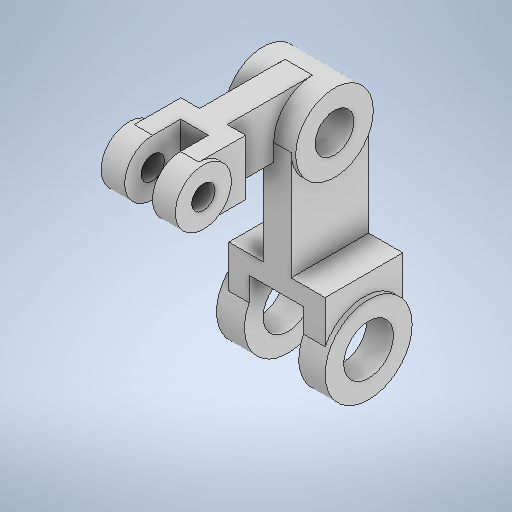
# Autodesk Inventor part: Sólido 2
Saved by Autodesk Inventor 2025 (Build 290162000, 162)
## iProperties
Created: 2024-04-28
Part Number: Sólido 2
Material: Generic
Document SubType Name: Modeling
Designer: kaike
Density: 1 g/cm^3
Appearance: Default
Author: kaike
Autodesk Inventor part; units mm, degrees
ref_plane "YZ Plane" through (0, 0, 0) normal (1, 0, 0) x (0, 1, 0)
ref_plane "XZ Plane" through (0, 0, 0) normal (0, 1, 0) x (-1, 0, 0)
sketch "Sketch1" plane through (0, 0, 0) normal (0, 0, 1) x (1, 0, 0)
  line L0 (31, 0) -> (31, 12)
  line L1 (31, 12) -> (9, 12)
  line L2 (9, 12) -> (9, 82)
  line L3 (31, 0) -> (17, 0)
  line L4 (17, 0) -> (0, 0)
  line L5 (9, 82) -> (0, 82)
  line L6 (-31, 0) -> (-31, 12)
  line L7 (-31, 12) -> (-9, 12)
  line L8 (-9, 12) -> (-9, 82)
  line L9 (-31, 0) -> (-17, 0)
  line L10 (-17, 0) -> (0, 0)
  line L11 (-9, 82) -> (0, 82)
  point P0 (0, 0)
  dimension "d7" = 14
  dimension "d8" = 17
  dimension "d10" = 70
  dimension "d11" = 22
  dimension "d12" = 12
  dimension "d13" = 18
  constraints: 24 end point, 2 horizontal
  measures "d7" distance of L0.start L3.end
  measures "d8" distance of L3.end L4.end
  measures "d10" distance of L8.start L11.start
  measures "d11" distance of L0.end L1.end
  measures "d12" distance of L0.start L0.end
  measures "d13" distance of L11.start L2.end
extrude "Extrusion1" add sketch "Sketch1" along normal mid plane 50
sketch "Sketch2" plane through (31, 0, 25) normal (1, 0, 0) x (0, 0, -1)
  line L0 (50, 82) -> (0, 82) projected
  circle A0 centre (25, -28) radius 28
  point P0 (25, 0)
  dimension "d17" = 56
  constraints: 1 centre point
  measures "d17" diameter of A0
extrude "Extrusion2" add sketch "Sketch2" along normal blind 3
sketch "Sketch3" plane through (31, 0, 25) normal (-1, 0, 0) x (0, 0, 1)
  arc A0 (-53, -28) -> (-25, 0) centre (-25, -28) ccw projected
  circle A1 centre (-25, -28) radius 28
  point P0 (-25, 0)
  constraints: 1 centre point, 1 coincident
extrude "Extrusion3" add sketch "Sketch3" along normal blind 67
sketch "Sketch5" plane through (9, 12, 25) normal (1, 0, 0) x (0, 0, -1)
  line L0 (50, 70) -> (0, 70) projected
  circle A0 centre (25, 70) radius 25
  point P0 (25, -12)
  dimension "d24" = 50
  constraints: 1 centre point, 1 midpoint
  measures "d24" diameter of A0
extrude "Extrusion5" add sketch "Sketch5" along normal blind 3
sketch "Sketch6" plane through (9, 12, 25) normal (-1, 0, 0) x (0, 0, 1)
  arc A0 (0, 70) -> (-50, 70) centre (-25, 70) ccw projected
  circle A1 centre (-25, 70) radius 25
  point P0 (-25, -12)
  point P1 (0, 70)
  constraints: 1 centre point, 1 coincident
extrude "Extrusion6" add sketch "Sketch6" along normal blind 43
sketch "Sketch7" plane through (-31, 12, 25) normal (0, 1, 0) x (1, 0, 0)
  point P0 (31, 25)
ref_plane "Work Plane1" through (12, 107, 55) normal (0, 1, 0) x (1, 0, 0)
sketch "Sketch10" plane through (12, 107, 55) normal (0, 1, 0) x (1, 0, 0)
  line L0 (-2.3312, -30.1107) -> (-2.219, -0.0002)
  line L1 (-2.219, -0.0002) -> (-14.1262, -0.0002)
  line L2 (-2.3312, -30.1107) -> (-14.238, -30.0664)
  line L3 (-44.0784, -29.9553) -> (-43.9668, 0.0445)
  line L4 (-43.9668, 0.0445) -> (-31.9669, -0.0002)
  line L5 (-44.0784, -29.9553) -> (-32.1716, -29.9996)
  line L6 (-14.1259, 55) -> (-31.9669, 55)
  line L7 (-2.219, 29.9997) -> (52.781, 29.9997) construction
  line L8 (-31.9669, -0.0002) -> (-31.9669, 55)
  line L9 (-14.1259, 55) -> (-14.1262, -0.0002)
  line L10 (-32.1716, -29.9996) -> (-14.238, -30.0664)
  constraints: 22 end point, 1 collinear, 1 horizontal, 1 perpendicular, 1 vertical
extrude "Extrusion8" add sketch "Sketch10" against normal blind 36
sketch "Sketch12" plane through (12, 82, 0) normal (1, 0, 0) x (0, 0, -1)
  circle A0 centre (0, 0) radius 12.5
  point P0 (0, -82)
  dimension "d48" = 25
  constraints: 1 centre point, 1 coincident
  measures "d48" diameter of A0
sketch "Sketch13" plane through (34, -28, 0) normal (1, 0, 0) x (0, 0, -1)
  circle A0 centre (0, 0) radius 16
  point P0 (0, 28)
  dimension "d49" = 32
  constraints: 1 centre point, 1 coincident
  measures "d49" diameter of A0
sketch "Sketch15" plane through (9.6688, 71, 85.1107) normal (1, 0, 0.0037) x (0.0037, 0, -1)
  line L0 (-0.0001, 36) -> (-0.0001, 0) projected
  circle A0 centre (-0.0001, 18) radius 18
  point P0 (85.0741, -71)
  constraints: 1 midpoint, 1 vertical alignment, 2 other
extrude "Extrusion9" add sketch "Sketch15" along normal blind 3
sketch "Sketch16" plane through (12.6688, 89, 85.1219) normal (1, 0, 0.0037) x (0.0037, 0, -1)
  circle A0 centre (0, 0) radius 18
  point P0 (85.0741, -89)
  constraints: 1 centre point
extrude "Extrusion10" add sketch "Sketch16" against normal blind 48
sketch "Sketch17" plane through (12, 107, 55) normal (0, 1, 0) x (1, 0, 0)
  line L0 (-32.1046, -11.9997) -> (-14.171, -12.0665) projected
  line L1 (-32.1046, -11.9997) -> (-32.1046, -64.3994)
  line L2 (-32.1046, -64.3994) -> (-14.171, -64.3994)
  line L3 (-14.171, -64.3994) -> (-14.171, -12.0665)
  line L4 (-14.171, -12.0665) -> (-32.1046, -11.9997)
  point P0 (-12, 55)
  constraints: 8 end point, 2 perpendicular, 1 collinear, 1 vertical
extrude "Extrusion11" cut sketch "Sketch17" against normal blind 48
sketch "Sketch18" plane through (12.6688, 89, 85.1219) normal (1, 0, 0.0037) x (0.0037, 0, -1)
  circle A0 centre (0, 0) radius 7.5
  point P0 (85.0741, -89)
  dimension "d56" = 15
  constraints: 1 centre point
  measures "d56" diameter of A0
extrude "Extrusion12" cut sketch "Sketch18" against normal blind 70
extrude "Extrusion13" cut sketch "Sketch12" against normal blind 70
extrude "Extrusion14" cut sketch "Sketch13" against normal blind 70
sketch "Sketch19" plane through (31, 0, 25) normal (1, 0, 0) x (0, 0, -1)
  line L0 (50, 12) -> (0, 12) projected
  line L1 (0, 12) -> (0, -21.7285)
  line L2 (0, -21.7285) -> (50, -21.7285)
  line L3 (50, -21.7285) -> (50, 12)
  line L4 (50, 12) -> (0, 12)
  point P0 (25, 0)
  constraints: 8 end point, 3 perpendicular, 1 vertical
extrude "Extrusion15" add sketch "Sketch19" against normal blind 62
sketch "Sketch20" plane through (34, -28, 0) normal (1, 0, 0) x (0, 0, -1)
  circle A0 centre (0, 0) radius 16
  point P0 (0, 28)
  constraints: 1 centre point
extrude "Extrusion16" cut sketch "Sketch20" against normal blind 70
sketch "Sketch21" plane through (0, 0, 25) normal (0, 0, 1) x (1, 0, 0)
  line L0 (0, 0) -> (17, 0)
  line L1 (17, 0) -> (17, -69.3639)
  line L2 (17, -69.3639) -> (-1, -69.3639)
  line L3 (-1, -69.3639) -> (-18, -69.3639)
  line L4 (-18, -69.3639) -> (-18, 0)
  line L5 (-18, 0) -> (0, 0)
  dimension "d67" = 17
  dimension "d68" = 17
  constraints: 12 end point, 4 perpendicular, 2 point on line, 1 horizontal
  measures "d67" distance of L0.start L0.end
  measures "d68" distance of L2.end L3.end
extrude "Extrusion17" cut sketch "Sketch21" along normal mid plane 150
body "Solid1"
